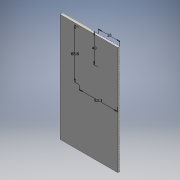
# Autodesk Inventor part: plate
Saved by Autodesk Inventor 2016 (Build 200138000, 138)
## iProperties
Created: 2018-07-05
Part Number: plate
Material: Generic
Document SubType Name: Modeling
Designer: andrew
Density: 1 g/cm^3
Appearance: Default
Author: andrew
Autodesk Inventor part; units mm, degrees
ref_plane "YZ Plane" through (0, 0, 0) normal (1, 0, 0) x (0, 1, 0)
ref_plane "XZ Plane" through (0, 0, 0) normal (0, 1, 0) x (-1, 0, 0)
ref_plane "XY Plane" through (0, 0, 0) normal (0, 0, 1) x (1, 0, 0)
sketch "Sketch1" plane through (0, 0, 0) normal (0, 1, 0) x (-1, 0, 0)
  line L0 (-40, 75) -> (40, 75)
  line L1 (40, 75) -> (40, -75)
  line L2 (40, -75) -> (-40, -75)
  line L3 (-40, -75) -> (-40, 75)
  line L4 (-40, 75) -> (40, -75) construction
  line L5 (40, 75) -> (-40, -75) construction
  point P0 (0, 0)
  dimension "d0" = 80
  dimension "d1" = 150
  constraints: 12 end point, 2 midpoint, 2 parallel, 1 horizontal, 1 perpendicular
  measures "d0" distance of L1.end L2.end
  measures "d1" distance of L0.end L1.end
extrude "Extrusion1" add sketch "Sketch1" along normal blind 3
sketch "Sketch2" plane through (0, 3, 0) normal (0, 1, 0) x (1, 0, 0)
  line L0 (-40, -75) -> (40, -75) construction
  line L1 (0, -75) -> (0, 75) construction
  line L2 (40, 75) -> (-40, 75) construction
  line L3 (40, -75) -> (40, 75) construction
  line L4 (40, 0) -> (-40, 0) construction
  line L5 (-40, 75) -> (-40, -75) construction
  line L6 (0, -75) -> (40, -75) construction
  line L7 (40, -75) -> (10, -75) construction
  line L8 (10, -75) -> (10, -35) construction
  line L9 (36.65, -69.3) -> (-16.65, -69.3) construction
  line L10 (-16.65, -69.3) -> (-16.65, -0.7) construction
  line L11 (-16.65, -0.7) -> (36.65, -0.7) construction
  line L12 (36.65, -0.7) -> (36.65, -69.3) construction
  line L13 (36.65, -69.3) -> (-16.65, -0.7) construction
  line L14 (-16.65, -69.3) -> (36.65, -0.7) construction
  point P0 (0, 0)
  dimension "d4" = 30
  dimension "d5" = 40
  dimension "d6" = 53.3
  dimension "d7" = 68.6
  constraints: 22 end point, 6 midpoint, 2 parallel, 2 perpendicular, 1 collinear, 1 horizontal, 1 point on line
  measures "d4" distance of L0.end L7.end
  measures "d5" distance of L7.end L8.end
  measures "d6" distance of L10.end L11.end
  measures "d7" distance of L9.end L10.end
body "Solid1"
